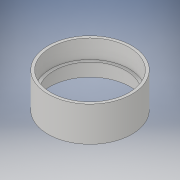
# Autodesk Inventor part: Skirt
Saved by Autodesk Inventor 2017 (Build 210142000, 142)
## iProperties
Created: 2016-07-19
Part Number: Skirt
Material: Generic
Document SubType Name: Modeling
Designer: Bill
Density: 1 g/cm^3
Appearance: Default
Author: Bill
Autodesk Inventor part; units mm, degrees
ref_plane "YZ Plane" through (0, 0, 0) normal (1, 0, 0) x (0, 1, 0)
ref_plane "XZ Plane" through (0, 0, 0) normal (0, 1, 0) x (-1, 0, 0)
ref_plane "XY Plane" through (0, 0, 0) normal (0, 0, 1) x (1, 0, 0)
sketch "Sketch1" plane through (0, 0, 0) normal (0, 0, 1) x (1, 0, 0)
  line L0 (-85.725, -25.252) -> (-82.55, -25.252)
  line L1 (-82.55, -25.252) -> (-73.7023, 7.768)
  line L2 (-73.7023, 7.768) -> (-80.0523, 7.768)
  line L3 (-80.0523, 7.768) -> (-80.0523, 45.868)
  line L4 (-80.0523, 45.868) -> (-85.725, 45.868)
  line L5 (-85.725, 45.868) -> (-85.725, -25.252)
  line L6 (0, -39.476) -> (0, 60.092) projected
  point P0 (0, 0)
  dimension "d0" = 3.175
  dimension "d2" = 105
  dimension "d3" = 82.55
  dimension "d4" = 6.35
  dimension "d5" = 71.12
  dimension "d6" = 38.1
  dimension "d7" = 5.6727
  dimension "d10" = 73.7023
  constraints: 12 end point, 2 perpendicular, 1 horizontal, 1 parallel, 1 vertical
  measures "d0" distance of L0.start L0.end
  measures "d2" angle of L0 L1
  measures "d3" horizontal distance of point (0, 0) L0.end
  measures "d4" distance of L1.end L2.end
  measures "d5" distance of L4.end L0.start
  measures "d6" distance of L2.end L3.end
  measures "d7" distance of L3.end L4.end
  measures "d10" distance from line of L6 L1.end
revolve "Revolution1" add sketch "Sketch1" angle 360 about axis through (0, -10, 0) along (0, 1, 0)
body "Solid1"
